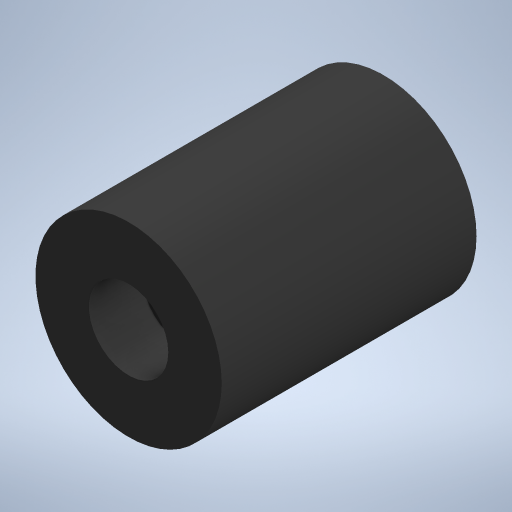
# Autodesk Inventor part: Cilindro_caucho
Saved by Autodesk Inventor 2024 (Build 280153000, 153)
## iProperties
Created: 2023-07-06
Part Number: Cilindro_caucho
Material: Caucho
Document SubType Name: Modeling
Designer: Arthur
Density: 0.93 g/cm^3
Appearance: Caucho - Negro
Author: Arthur
Autodesk Inventor part; units mm, degrees
ref_plane "YZ Plane" through (0, 0, 0) normal (1, 0, 0) x (0, 1, 0)
ref_plane "XZ Plane" through (0, 0, 0) normal (0, 1, 0) x (-1, 0, 0)
ref_plane "XY Plane" through (0, 0, 0) normal (0, 0, 1) x (1, 0, 0)
sketch "Boceto1" plane through (0, 0, 0) normal (0, 0, 1) x (1, 0, 0)
  circle A0 centre (0, 0) radius 4.75
  dimension "d0" = 9.5
  constraints: 1 centre point, 1 coincident
  measures "d0" diameter of A0
extrude "Extrusión1" add sketch "Boceto1" along normal blind 13
sketch "Boceto2" plane through (0, 0, 13) normal (0, 0, 1) x (1, 0, 0)
  circle A0 centre (0, 0) radius 2.025
  dimension "d3" = 4.05
  constraints: 1 centre point, 1 coincident
  measures "d3" diameter of A0
extrude "Extrusión2" cut sketch "Boceto2" against normal blind 11
sketch "Boceto3" plane through (0, 0, 0) normal (1, 0, 0) x (0, 1, 0)
  line L0 (2.025, 13) -> (2.025, 2) projected
  line L1 (2.025, 2) -> (2.025, 6)
  line L2 (1.25, 6) -> (-1.25, 6)
  line L3 (-2.025, 13) -> (-2.025, 2) projected
  line L4 (0, 6) -> (-1.25, 6)
  line L5 (0, 6) -> (1.25, 6)
  arc A0 (2.025, 6.775) -> (2.025, 5.225) centre (2.025, 6) ccw
  arc A1 (-2.025, 5.225) -> (-2.025, 6.775) centre (-2.025, 6) ccw
  line L6 (2.025, 6) -> (2.025, 10)
  line L7 (1.75, 10) -> (-1.75, 10)
  line L8 (0, 10) -> (-1.75, 10)
  line L9 (0, 10) -> (1.75, 10)
  arc A2 (2.025, 10.275) -> (2.025, 9.725) centre (2.025, 10) ccw
  arc A3 (-2.025, 9.725) -> (-2.025, 10.275) centre (-2.025, 10) ccw
  line L10 (-2.025, 2) -> (2.025, 2) projected
  line L11 (0, 2) -> (0, 13)
  line L12 (4.75, 13) -> (-4.75, 13) projected
  point P0 (0, 0)
  point P1 (2.025, 5.225)
  dimension "d7" = 4
  dimension "d8" = 1.25
  dimension "d9" = 1.25
  dimension "d10" = 4
  dimension "d11" = 1.75
  dimension "d12" = 1.75
  constraints: 18 end point, 12 point on circle, 11 point on line, 4 centre point, 4 midpoint, 2 coincident, 2 perpendicular
  measures "d7" distance of L1.start L1.end
  measures "d8" distance of L2.end L4.start
  measures "d9" distance of L2.start L4.start
  measures "d10" distance of L6.start L6.end
  measures "d11" distance of L7.end L8.start
  measures "d12" distance of L7.start L8.start
revolve "Revolución1" add sketch "Boceto3" angle 360 about axis through (0, 0, 2) along (0, 0, 1) contours L0 A2 | A3 L3 | L0 A0 | A1 L3
